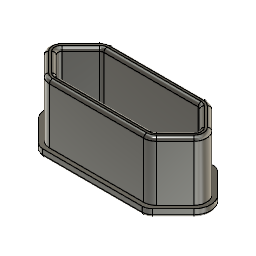
EuroDust (Autodesk Fusion 360 design; units mm, degrees)
Autodesk Fusion 360 part; units mm, degrees
note: some values were not read from the file. Chosen so that the rebuilt part matches the saved one: which face or edge a step refers to. Set by a fixed rule: which sketch regions a step uses.
sketch "Sketch1" plane through (0, 0, 0) normal (0, 0, 1) x (1, 0, 0)
  line L0 (-11.3672, 7.5) -> (11.1475, 7.5)
  line L1 (13.2688, 6.6213) -> (17.7688, 2.1213)
  line L2 (17.7688, -2.1213) -> (13.2688, -6.6213)
  line L3 (11.1475, -7.5) -> (-11.3672, -7.5)
  line L4 (-13.4885, -6.6213) -> (-17.9885, -2.1213)
  line L5 (-17.9885, 2.1213) -> (-13.4885, 6.6213)
  line L6 (-20.1099, 0) -> (19.8901, 0) construction
  arc A0 (-17.9885, 2.1213) -> (-17.9885, -2.1213) centre (-15.8672, 0) ccw
  arc A1 (17.7688, -2.1213) -> (17.7688, 2.1213) centre (15.6475, 0) ccw
  arc A2 (-11.3672, 7.5) -> (-13.4885, 6.6213) centre (-11.3672, 4.5) ccw
  arc A3 (13.2688, 6.6213) -> (11.1475, 7.5) centre (11.1475, 4.5) ccw
  arc A4 (11.1475, -7.5) -> (13.2688, -6.6213) centre (11.1475, -4.5) ccw
  arc A5 (-13.4885, -6.6213) -> (-11.3672, -7.5) centre (-11.3672, -4.5) ccw
  dimension "d1" = 135
  dimension "d2" = 135
  dimension "d4" = 135
  dimension "d5" = 135
  dimension "d6" = 40
  dimension "d7" = 15
  dimension "d14" = 3
  dimension "d15" = 3
  dimension "d37" = 3
  dimension "d41" = 3
  dimension "d42" = 3
  dimension "d43" = 3
  dimension "d44" = 7.5
  dimension "d45" = 15
  measures "d1" angle of L0 L1
  measures "d2" angle of L3 L4
  measures "d4" angle of L0 L5
  measures "d5" angle of L2 L3
  measures "d6" distance of L6.end L6.start
  measures "d7" distance of L0 L3
  measures "d14" radius of A0
  measures "d15" radius of A1
  measures "d37" radius of A2
  measures "d41" radius of A4
  measures "d42" radius of A5
  measures "d43" radius of A3
  measures "d44" distance of origin L3
  measures "d45" distance of L0 L3
extrude "Extrude1" add sketch "Sketch1" along normal blind 14 makes body 1
sketch "Sketch2" plane through (0, 0, 0) normal (0, 0, -1) x (1, 0, 0)
  line L0 (-13.4885, 6.6213) -> (-17.9885, 2.1213)
  line L1 (-17.9885, -2.1213) -> (-13.4885, -6.6213)
  line L2 (-11.3672, -7.5) -> (11.1475, -7.5)
  line L3 (13.2688, -6.6213) -> (17.7688, -2.1213)
  line L4 (17.7688, 2.1213) -> (13.2688, 6.6213)
  line L5 (11.1475, 7.5) -> (-11.3672, 7.5)
  line L6 (-11.9885, -8.5) -> (11.7688, -8.5)
  line L7 (13.5366, -7.7678) -> (18.4759, -2.8284)
  line L8 (18.4759, 2.8284) -> (13.5366, 7.7678)
  line L9 (11.7688, 8.5) -> (-11.9885, 8.5)
  line L10 (-13.7563, 7.7678) -> (-18.6956, 2.8284)
  line L11 (-18.6956, -2.8284) -> (-13.7563, -7.7678)
  arc A0 (-17.9885, 2.1213) -> (-17.9885, -2.1213) centre (-15.8672, 0) ccw
  arc A1 (17.7688, -2.1213) -> (17.7688, 2.1213) centre (15.6475, 0) ccw
  arc A2 (-18.6956, 2.8284) -> (-18.6956, -2.8284) centre (-15.8672, 0) ccw
  arc A3 (18.4759, -2.8284) -> (18.4759, 2.8284) centre (15.6475, 0) ccw
  arc A4 (-13.4885, -6.6213) -> (-11.3672, -7.5) centre (-11.3672, -4.5) ccw
  arc A5 (11.1475, -7.5) -> (13.2688, -6.6213) centre (11.1475, -4.5) ccw
  arc A6 (13.2688, 6.6213) -> (11.1475, 7.5) centre (11.1475, 4.5) ccw
  arc A7 (-11.3672, 7.5) -> (-13.4885, 6.6213) centre (-11.3672, 4.5) ccw
  arc A8 (-13.7563, -7.7678) -> (-11.9885, -8.5) centre (-11.9885, -6) ccw
  arc A9 (11.7688, -8.5) -> (13.5366, -7.7678) centre (11.7688, -6) ccw
  arc A10 (13.5366, 7.7678) -> (11.7688, 8.5) centre (11.7688, 6) ccw
  arc A11 (-11.9885, 8.5) -> (-13.7563, 7.7678) centre (-11.9885, 6) ccw
  dimension "d16" = 4
  dimension "d17" = 4
  dimension "d33" = 1
  dimension "d34" = 1
  dimension "d38" = 2.5
  measures "d16" radius of A2
  measures "d17" radius of A3
  measures "d33" distance of L5 L9
  measures "d34" distance of L2 L6
  measures "d38" radius of A8
extrude "Extrude2" add sketch "Sketch2" along normal blind 2 contours L0 L1 L2 L3 L4 L5 A0 A1 A4 A5 A6 A7 | L6 L7 L8 L9 L10 L11 A2 A3 A8 A9 A10 A11 bodies 1
shell "Shell1" thickness 2 removed faces 1 at (-3.8623, 2.5, 14) on bodies 1
sketch "Sketch4" plane through (0, 0, 14) normal (0, 0, 1) x (-1, 0, 0)
  line L0 (-16.3546, 0.7071) -> (-11.8546, 5.2071)
  line L1 (16.5743, -0.7071) -> (12.0743, -5.2071)
  line L2 (11.3672, -5.5) -> (-11.1475, -5.5)
  line L3 (-11.8546, -5.2071) -> (-16.3546, -0.7071)
  line L4 (-13.2688, 6.6213) -> (-17.7688, 2.1213)
  arc A0 (-17.7688, 2.1213) -> (-17.7688, -2.1213) centre (-15.6475, 0) ccw
  line L5 (-17.7688, -2.1213) -> (-13.2688, -6.6213)
  line L6 (-11.1475, -7.5) -> (11.3672, -7.5)
  line L7 (13.4885, -6.6213) -> (17.9885, -2.1213)
  arc A1 (17.9885, -2.1213) -> (17.9885, 2.1213) centre (15.8672, 0) ccw
  line L8 (11.3672, 7.5) -> (-11.1475, 7.5)
  line L9 (8.3672, -7.5) -> (-10.2688, -7.5)
  line L10 (-10.2688, -7.5) -> (-10.2688, -5.5)
  line L11 (-10.2688, -5.5) -> (8.3672, -5.5)
  line L12 (8.3672, -5.5) -> (8.3672, -7.5)
  line L13 (8.3672, 5.5) -> (-10.2688, 5.5)
  line L14 (-10.2688, 5.5) -> (-10.2688, 7.5)
  line L15 (-10.2688, 7.5) -> (8.3672, 7.5)
  line L16 (8.3672, 7.5) -> (8.3672, 5.5)
  line L17 (-11.1475, 5.5) -> (11.3672, 5.5)
  arc A2 (11.3672, -5.5) -> (12.0743, -5.2071) centre (11.3672, -4.5) ccw
  arc A3 (-11.8546, -5.2071) -> (-11.1475, -5.5) centre (-11.1475, -4.5) ccw
  arc A4 (-11.1475, 5.5) -> (-11.8546, 5.2071) centre (-11.1475, 4.5) ccw
  arc A5 (12.0743, 5.2071) -> (11.3672, 5.5) centre (11.3672, 4.5) ccw
  arc A6 (13.4885, 6.6213) -> (11.3672, 7.5) centre (11.3672, 4.5) ccw
  arc A7 (-11.1475, 7.5) -> (-13.2688, 6.6213) centre (-11.1475, 4.5) ccw
  arc A8 (-13.2688, -6.6213) -> (-11.1475, -7.5) centre (-11.1475, -4.5) ccw
  arc A9 (11.3672, -7.5) -> (13.4885, -6.6213) centre (11.3672, -4.5) ccw
  arc A10 (16.5743, -0.7071) -> (16.5743, 0.7071) centre (15.8672, 0) ccw
  arc A11 (-16.3546, 0.7071) -> (-16.3546, -0.7071) centre (-15.6475, 0) ccw
  dimension "d35" = 3
  dimension "d36" = 3
  measures "d35" distance of L6.end L12
  measures "d36" distance of L5.end L10
fillet "Fillet1" radius 0.75 12 edges at (-12.9452, 8.3097, -2) (-16.226, 5.2981, -2) (-0.1099, 8.5, -2) (12.7255, 8.3097, -2) (16.0063, 5.2981, -2) (19.6475, 0, -2) (16.0063, -5.2981, -2) (12.7255, -8.3097, -2) (-0.1099, -8.5, -2) (-12.9452, -8.3097, -2) (-16.226, -5.2981, -2) (-19.8672, 0, -2) on bodies 1
fillet "Fillet2" radius 0.75 24 edges at (-0.1099, 7.5, 14) (12.2956, 7.2716, 14) (15.5188, 4.3713, 14) (18.6475, 0, 14) (15.5188, -4.3713, 14) (12.2956, -7.2716, 14) (-0.1099, -7.5, 14) (-12.5153, -7.2716, 14) (-15.7385, -4.3713, 14) (-18.8672, 0, 14) (-15.7385, 4.3713, 14) (-12.5153, 7.2716, 14) (-14.3243, 2.9571, 14) (-11.7499, 5.4239, 14) (-0.1099, 5.5, 14) (11.5302, 5.4239, 14) (14.1046, 2.9571, 14) (16.6475, 0, 14) (14.1046, -2.9571, 14) (11.5302, -5.4239, 14) (-0.1099, -5.5, 14) (-11.7499, -5.4239, 14) (-14.3243, -2.9571, 14) (-16.8672, 0, 14) on bodies 1
copy_body "Body->Comp1" bodies 1 removing the originals makes body 2 in component "EuroDust"
component "EuroDust" placed x (1, 0, 0) y (0, 1, 0) z (0, 0, 1) at (0, 0, 0)
equation "d1 = 90 deg + 45 deg"
named bodies: "EuroDust"
